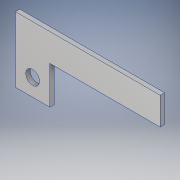
# Autodesk Inventor part: Spreader Flag
Saved by Autodesk Inventor 2018 (Build 220112000, 112)
## iProperties
Created: 2013-10-19
Part Number: Spreader Flag
Material: Aluminum 6061
Document SubType Name: Modeling
Designer: Gabriel Smolnycki
Mass: 2.34054 g
Surface Area: 11.36 cm^2
Volume: 0.866867 cm^3
Density: 2.7 g/cm^3
Appearance: Aluminum - Flat
Sending System: SolidWorks 2017
Last Author: Gabriel Smolnycki
Last Saved: 2017-09-14
Author: Gabriel Smolnycki
Autodesk Inventor part; units mm, degrees
ref_plane "YZ Plane" through (0, 0, 0) normal (1, 0, 0) x (0, 1, 0)
ref_plane "XZ Plane" through (0, 0, 0) normal (0, 1, 0) x (-1, 0, 0)
ref_plane "XY Plane" through (0, 0, 0) normal (0, 0, 1) x (1, 0, 0)
sketch "Sketch1" plane through (0, 0, 0) normal (0, 0, 1) x (1, 0, 0)
  line L0 (0, 0) -> (10, 0)
  line L1 (0, 19) -> (42, 19)
  line L2 (10, 11) -> (10, 0)
  line L3 (42, 11) -> (10, 11)
  line L4 (0, 19) -> (0, 0)
  line L5 (42, 11) -> (42, 19)
  constraints: 12 end point, 3 horizontal, 3 vertical
extrude "Extrusion1" add sketch "Sketch1" along normal blind 1.27
sketch "Sketch2" plane through (0, 0, 0) normal (0, 0, 1) x (1, 0, 0)
  point P0 (5, 5)
hole "Hole1" at (5, 5, 0) direction (0, 0, 1) diameter 4 depth 1.27 tip angle 118
body "Solid3"
